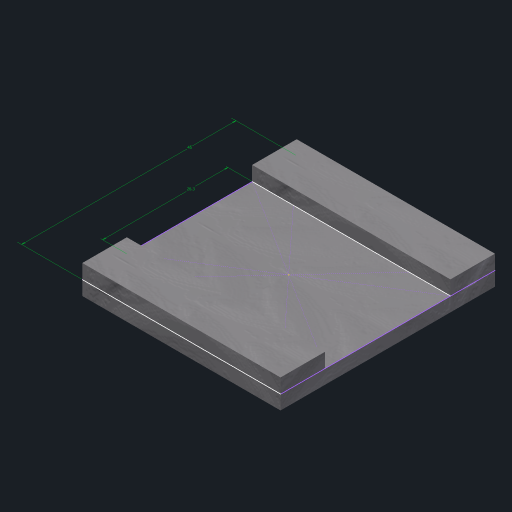
# Autodesk Inventor part: ESPACIADOR_CREMALLERA
Saved by Autodesk Inventor 2024.3 (Build 283343000, 343)
## iProperties
Created: 2024-07-19
Part Number: ESPACIADOR_CREMALLERA
Material: Steel, Mild, Welded
Document SubType Name: Modeling
Designer: Niler
Density: 7.85 g/cm^3
Appearance: Weld - Steel Mild
Author: Niler
Autodesk Inventor part; units mm, degrees
ref_plane "YZ Plane" through (0, 0, 0) normal (1, 0, 0) x (0, 1, 0)
ref_plane "XZ Plane" through (0, 0, 0) normal (0, 1, 0) x (-1, 0, 0)
ref_plane "XY Plane" through (0, 0, 0) normal (0, 0, 1) x (1, 0, 0)
sketch "Sketch1" plane through (0, 0, 0) normal (0, 1, 0) x (-1, 0, 0)
  line L0 (-20.8041, 22.5) -> (20.8041, 22.5)
  line L1 (20.8041, 22.5) -> (20.8041, -22.5)
  line L2 (20.8041, -22.5) -> (-20.8041, -22.5)
  line L3 (-20.8041, -22.5) -> (-20.8041, 22.5)
  line L4 (-20.8041, 22.5) -> (20.8041, -22.5) construction
  line L5 (20.8041, 22.5) -> (-20.8041, -22.5) construction
  line L6 (-20.8041, -13.15) -> (20.8041, -13.15)
  line L7 (20.8041, -13.15) -> (20.8041, 13.15)
  line L8 (20.8041, 13.15) -> (-20.8041, 13.15)
  line L9 (-20.8041, 13.15) -> (-20.8041, -13.15)
  line L10 (-20.8041, -13.15) -> (20.8041, 13.15) construction
  line L11 (20.8041, -13.15) -> (-20.8041, 13.15) construction
  point P0 (0, 0)
  dimension "d0" = 26.3
  dimension "d1" = 45
  constraints: 24 end point, 4 midpoint, 4 parallel, 2 horizontal, 2 perpendicular, 1 point on line
  measures "d0" distance between parallel lines of L6 L8
  measures "d1" distance between parallel lines of L2 L0
extrude "Extrusion1" add sketch "Sketch1" along normal blind 3 contours L0 L1 L8 L3 | L6 L1 L2 L3
extrude "Extrusion2" add sketch "Sketch1" against normal blind 3
body "Solid1"
